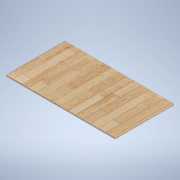
# Autodesk Inventor part: PlywoodBasePlate17_25x32_03x0_5inches
Saved by Autodesk Inventor 2022.2 (Build 262287000, 287)
## iProperties
Created: 2022-01-23
Part Number: PlywoodBasePlate17_25x32_03x0_5inches
Material: Wood (Maple)
Document SubType Name: Modeling
Designer: robst
Density: 0.67 g/cm^3
Appearance: Natural Maple - Glossy Dark Tint
Author: robst
Autodesk Inventor part; units mm, degrees
ref_plane "YZ Plane" through (0, 0, 0) normal (1, 0, 0) x (0, 1, 0)
ref_plane "XZ Plane" through (0, 0, 0) normal (0, 1, 0) x (-1, 0, 0)
ref_plane "XY Plane" through (0, 0, 0) normal (0, 0, 1) x (1, 0, 0)
sketch "Sketch2" plane through (0, 0, 0) normal (0, 1, 0) x (-1, 0, 0)
  line L0 (406.781, 219.075) -> (-406.781, 219.075)
  line L1 (-406.781, 219.075) -> (-406.781, -219.075)
  line L2 (-406.781, -219.075) -> (406.781, -219.075)
  line L3 (406.781, -219.075) -> (406.781, 219.075)
  line L4 (406.781, 219.075) -> (-406.781, -219.075) construction
  line L5 (-406.781, 219.075) -> (406.781, -219.075) construction
  point P0 (0, 0)
  dimension "d0" = 813.562
  dimension "d1" = 438.15
  constraints: 12 end point, 2 midpoint, 2 parallel, 1 horizontal, 1 perpendicular
  measures "d0" distance of L0.start L0.end
  measures "d1" distance of L1.end L0.end
extrude "Extrusion1" add sketch "Sketch2" against normal blind 12.7
body "Solid1"
